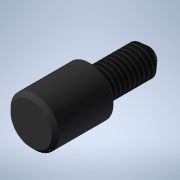
# Autodesk Inventor part: 8617.540_P4
Saved by Autodesk Inventor 2021 (Build 250183000, 183)
## iProperties
Created: 2026-08-04
Part Number: 8617.540_P4
Material: Generic
Catalog Web Link: www.3dfindit.com
Description: VX Teilmontageplatte - P4-VX Teilmontageplatte - P4
Vendor: RITTAL
Document SubType Name: Modeling
Designer: psAdmin
Manufacturer: RITTAL
Mass: 2.86776 g
Surface Area: 12.3343 cm^2
Volume: 2.86776 cm^3
Density: 1 g/cm^3
Appearance: PSOLRGB-176-176-176
Category: PARTsolutions
Company: RITTAL
Title: 8617.540_P4
Author: Cadenas PARTsolutions
Comments: VX Teilmontageplatte - P4
PSOL_IDENT_0: {$CADENAS_DATA/23d-libs/rittal/sys_zub/innenausbau/montageplatten/parts/teilmontageplatten_m51_p4.pr
PSOL_IDENT_1: j},181 {VTYP=3D},{NB=8617.540_P4},{LINA=8617.540_P4},{NN=VX Teilmontageplatte - P4},{DATE=16.02.2026
PSOL_IDENT_2: 20:13:30},{GEOMDATE=11.04.2025 11:24:24},{VERSION=},{LINEID=40},{WBVAR=},{WBNUMERIC=}  {NB=8617.540
PSOL_IDENT_3: _P4},{LINA=8617.540_P4},{KT=DUMMY},{BEST=8617.540},{INFO=PDF Katalog},{BEZ1=VX Teilmontageplatte},{B
PSOL_IDENT_4: EZ2=für neues Großschranksystem},{B=600},{BB=499},{H=800},{HH=699},{SB=600},{SH=800},{AB=600 x 800},
PSOL_IDENT_5: {VE=1},{VERS=4},{INFOPAGE=hb35_s707},{INFOPATH=hb35_s707_en.pdf},{CNSECLASS51=27-18-92-31},{CNSECLAS
PSOL_IDENT_6: S70=27-40-92-16},{CNSECLASS80=27-40-92-16},{CNSETIM40=EC000213},{BEZ3=},{DETAIL=1},{ADDGEO=1},{GEW=9
PSOL_IDENT_7: ,22},{CNSETIM80=EC000213},{CNSETIM90=EC000213},{CNSECLASS60=27-40-92-16},{UNSPSC=31-26-15-02}
NB: 8617.540_P4
NN: VX Teilmontageplatte - P4
NT: VX Teilmontageplatte - P4
NBSYN: $BEST._P4
LINA: 8617.540_P4
CATALOG: Rittal
BEST: 8617.540
INFO: PDF Katalog
BEZ1: VX Teilmontageplatte
BB: 499
HH: 699
SB: 600
SH: 800
CNSECLASS70: 27-40-92-16
CNSECLASS80: 27-40-92-16
GEW: 9,22
CNSETIM80: EC000213
CNSETIM90: EC000213
CNSECLASS60: 27-40-92-16
UNSPSC: 31-26-15-02
SUPPLIER: RITTAL
ARTICLENO: 8617.540_P4
BOMINFO: 8617.540_P4
CREATOR: CADENAS GmbH
Autodesk Inventor part; units mm, degrees
sketch "Sketch_1" plane through (0, 0, 0) normal (1, 0, 0) x (0, 0, -1)
  line L0 (12.5, 0) -> (-19, 0)
  line L1 (-19, 0) -> (-19, 5.5)
  line L2 (-19, 5.5) -> (-18, 6.5)
  line L3 (-18, 6.5) -> (-3.5, 6.5)
  line L4 (-3.5, 6.5) -> (-2.5, 5.5)
  line L5 (-2.5, 5.5) -> (-2.5, 4)
  line L6 (-2.5, 4) -> (10.5003, 4)
  line L7 (10.5003, 4) -> (12.5, 2.25)
  line L8 (12.5, 2.25) -> (12.5, 0)
  line L9 (12.5, 0) -> (-19, 0)
  constraints: 20 end point
revolve "Revolution1" add sketch "Sketch_1" angle 360 about axis through (0, 0, -12.5) along (0, 0, -1)
thread "Thread1" size "M8x1.25" class "6g" standard "ISO Metric profile" full length
ref_plane "P4_XY" through (0, 0, 0) normal (0, 0, 1) x (1, 0, 0)
ref_plane "P4_YZ" through (0, 0, 0) normal (1, 0, 0) x (0, 1, 0)
ref_plane "P4_ZX" through (0, 0, 0) normal (0, 1, 0) x (0, 0, 1)
body "Solid1"
